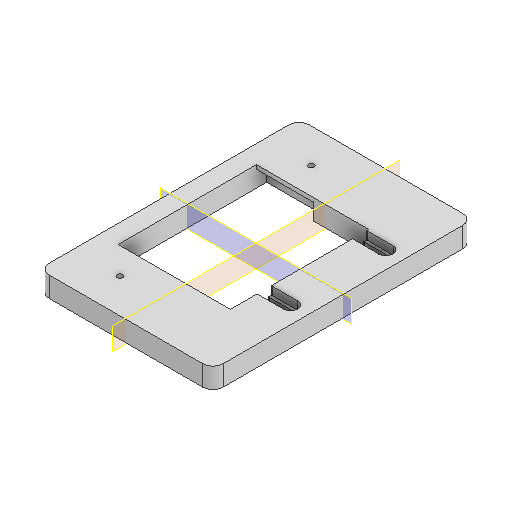
# Autodesk Inventor part: TIRFImager_base_v0
Saved by Autodesk Inventor 2022 (Build 260153000, 153)
## iProperties
Created: 2022-05-21
Part Number: TIRFImager_base_v0
Material: Generisch
Document SubType Name: Modeling
Designer: diederichbenedict
Density: 1 g/cm^3
Appearance: Vorgabe
Author: diederichbenedict
Autodesk Inventor part; units mm, degrees
ref_plane "YZ Plane" through (0, 0, 0) normal (1, 0, 0) x (0, 1, 0)
ref_plane "XZ Plane" through (0, 0, 0) normal (0, 1, 0) x (-1, 0, 0)
ref_plane "XY Plane" through (0, 0, 0) normal (0, 0, 1) x (1, 0, 0)
sketch "Skizze1" plane through (0, 0, 0) normal (0, 1, 0) x (-1, 0, 0)
  line L0 (-37.75, -63.9) -> (37.75, -63.9)
  line L1 (42.75, -58.9) -> (42.75, 58.9)
  line L2 (37.75, 63.9) -> (-37.75, 63.9)
  line L3 (-42.75, 58.9) -> (-42.75, -58.9)
  line L4 (-42.75, -63.9) -> (42.75, 63.9) construction
  line L5 (42.75, -63.9) -> (-42.75, 63.9) construction
  arc A0 (42.75, 58.9) -> (37.75, 63.9) centre (37.75, 58.9) ccw
  arc A1 (-37.75, 63.9) -> (-42.75, 58.9) centre (-37.75, 58.9) ccw
  arc A2 (-42.75, -58.9) -> (-37.75, -63.9) centre (-37.75, -58.9) ccw
  arc A3 (37.75, -63.9) -> (42.75, -58.9) centre (37.75, -58.9) ccw
  point P0 (0, 0)
  dimension "d0" = 85.5
  dimension "d1" = 127.8
  dimension "d2" = 5
  constraints: 12 end point, 8 point on circle, 8 point on line, 8 tangent, 4 centre point, 3 equal radius, 2 midpoint, 2 parallel, 1 horizontal, 1 perpendicular
  measures "d0" distance of L5.end L4.end
  measures "d1" distance of L4.end L5.start
  measures "d2" radius of A0
extrude "Extrusion1" add sketch "Skizze1" along normal blind 10
ref_plane "Arbeitsebene1" through (37.75, 0, 0) normal (0, 0, -1) x (-1, 0, 0)
ref_plane "Arbeitsebene2" through (0, 0, 58.9) normal (1, 0, 0) x (0, 0, -1)
sketch "Skizze2" plane through (0, 10, 0) normal (0, 1, 0) x (1, 0, 0)
  line L0 (-6.95, 38) -> (-32.75, 38) projected
  line L1 (-32.75, -38) -> (-6.95, -38) projected
  line L2 (-6.95, -38) -> (-6.95, -2.5) projected
  line L3 (-32.75, 38) -> (-32.75, -38) projected
  line L4 (-32.75, -38) -> (-6.95, -38)
  line L5 (-6.95, -38) -> (-6.95, 38)
  line L6 (-6.95, 38) -> (-32.75, 38)
  line L7 (-32.75, 38) -> (-32.75, -38)
  line L8 (-5.95, 39) -> (-5.95, -39)
  line L9 (-5.95, -39) -> (-33.75, -39)
  line L10 (-33.75, -39) -> (-33.75, 39)
  line L11 (-33.75, 39) -> (-5.95, 39)
  point P0 (0, 0)
  dimension "d5" = 1
  constraints: 16 end point, 4 parallel, 2 perpendicular, 1 horizontal, 3 other
  measures "d5" distance between parallel lines of L5 L8
extrude "Extrusion2" cut sketch "Skizze2" against normal through all contours L5 L2 L1 L3 L0 | L8 L9 L10 L11
ref_plane "Arbeitsebene3" through (-32.75, 5, -38) normal (0, 1, 0) x (0, 0, 1)
sketch "Skizze3" plane through (0, 10, 0) normal (0, 1, 0) x (1, 0, 0)
  line L0 (-5.95, -39) -> (-33.75, -39) projected
  line L1 (-33.75, -39) -> (-33.75, 39) projected
  line L2 (-33.75, 39) -> (-5.95, 39) projected
  line L3 (-5.95, 39) -> (-5.95, -39) projected
  arc A0 (-37.75, 63.9) -> (-42.75, 58.9) centre (-37.75, 58.9) ccw projected
  line L4 (-42.75, 58.9) -> (-42.75, -58.9) projected
  arc A1 (-42.75, -58.9) -> (-37.75, -63.9) centre (-37.75, -58.9) ccw projected
  line L5 (-37.75, -63.9) -> (37.75, -63.9) projected
  arc A2 (37.75, -63.9) -> (42.75, -58.9) centre (37.75, -58.9) ccw projected
  line L6 (42.75, -58.9) -> (42.75, 58.9) projected
  arc A3 (42.75, 58.9) -> (37.75, 63.9) centre (37.75, 58.9) ccw projected
  line L7 (37.75, 63.9) -> (-37.75, 63.9) projected
  line L8 (-33.75, -39) -> (-33.75, 39) projected
  line L9 (-5.95, 39) -> (-5.95, -39) projected
  line L10 (-33.75, -39) -> (-5.95, -39)
  line L11 (-5.95, -39) -> (-5.95, -34)
  line L12 (-5.95, -34) -> (-33.75, -34)
  line L13 (-33.75, -34) -> (-33.75, -39)
  line L14 (-33.75, 39) -> (-5.95, 39)
  line L15 (-5.95, 39) -> (-5.95, 34)
  line L16 (-5.95, 34) -> (-33.75, 34)
  line L17 (-33.75, 34) -> (-33.75, 39)
  point P0 (0, 0)
  point P1 (-5.95, 34)
  point P2 (-5.95, -34)
  dimension "d8" = 27.8
  dimension "d9" = 5
  dimension "d10" = 5
  constraints: 16 end point, 4 parallel, 2 horizontal, 2 perpendicular, 2 point on line
  measures "d8" distance of L12.end L11.end
  measures "d9" distance of L11.end L10.end
  measures "d10" distance of L14.end L15.end
extrude "Extrusion3" add sketch "Skizze3" against normal blind 1 contours L0 L1 L12 L3 | L16 L1 L2 L3
sketch "Skizze4" plane through (0, 0, 0) normal (0, -1, 0) x (1, 0, 0)
  line L0 (-33.75, 39) -> (-5.95, 39) projected
  line L1 (-5.95, 39) -> (-5.95, -39) projected
  line L2 (-5.95, -39) -> (-33.75, -39) projected
  line L3 (-33.75, -39) -> (-33.75, 39) projected
  arc A0 (-42.75, -58.9) -> (-37.75, -63.9) centre (-37.75, -58.9) ccw projected
  line L4 (37.75, -63.9) -> (-37.75, -63.9) projected
  arc A1 (37.75, -63.9) -> (42.75, -58.9) centre (37.75, -58.9) ccw projected
  line L5 (42.75, 58.9) -> (42.75, -58.9) projected
  arc A2 (42.75, 58.9) -> (37.75, 63.9) centre (37.75, 58.9) ccw projected
  line L6 (-37.75, 63.9) -> (37.75, 63.9) projected
  arc A3 (-37.75, 63.9) -> (-42.75, 58.9) centre (-37.75, 58.9) ccw projected
  line L7 (-42.75, -58.9) -> (-42.75, 58.9) projected
  line L8 (-5.95, -34) -> (-5.95, 34) projected
  line L9 (-5.95, 34) -> (21.3958, 34)
  line L10 (21.3958, 34) -> (21.3958, -34)
  line L11 (21.3958, -34) -> (-5.95, -34)
  line L12 (-5.95, -34) -> (-5.95, 34)
  line L13 (3.55, 7.5) -> (3.55, -8) projected
  point P0 (0, 0)
  point P1 (-5.95, -34)
  dimension "d14" = 5
  dimension "d15" = 5
  constraints: 8 end point, 2 parallel, 1 horizontal, 1 perpendicular, 1 point on line
  measures "d14" distance between parallel lines of L2 L11
  measures "d15" distance between parallel lines of L9 L0
extrude "Extrusion4" cut sketch "Skizze4" against normal through all contours L9 L10 L11 L1
sketch "Skizze5" plane through (0, 0, 0) normal (0, -1, 0) x (1, 0, 0)
  arc A0 (-42.75, -58.9) -> (-37.75, -63.9) centre (-37.75, -58.9) ccw projected
  line L0 (37.75, -63.9) -> (-37.75, -63.9) projected
  arc A1 (37.75, -63.9) -> (42.75, -58.9) centre (37.75, -58.9) ccw projected
  line L1 (42.75, 58.9) -> (42.75, -58.9) projected
  arc A2 (42.75, 58.9) -> (37.75, 63.9) centre (37.75, 58.9) ccw projected
  line L2 (-37.75, 63.9) -> (37.75, 63.9) projected
  arc A3 (-37.75, 63.9) -> (-42.75, 58.9) centre (-37.75, 58.9) ccw projected
  line L3 (-42.75, -58.9) -> (-42.75, 58.9) projected
  line L4 (-5.95, 34) -> (21.3958, 34) projected
  line L5 (21.3958, 34) -> (21.3958, -34) projected
  line L6 (21.3958, -34) -> (-5.95, -34) projected
  line L7 (-5.95, -34) -> (-5.95, -39) projected
  line L8 (-5.95, -39) -> (-33.75, -39) projected
  line L9 (-33.75, -39) -> (-33.75, 39) projected
  line L10 (-33.75, 39) -> (-5.95, 39) projected
  line L11 (-5.95, 39) -> (-5.95, 34) projected
  circle A4 centre (-19.85, -47) radius 1.4
  circle A5 centre (-19.85, 47) radius 1.4
  point P0 (0, 0)
  dimension "d18" = 2.8
  dimension "d19" = 2.8
  dimension "d20" = 8
  dimension "d21" = 8
  constraints: 2 centre point
  measures "d18" diameter of A4
  measures "d19" diameter of A5
  measures "d20" distance from line of L8 A4.centre
  measures "d21" distance from line of A5.centre L10
extrude "Extrusion5" cut sketch "Skizze5" against normal through all contours A4 | A5
sketch "Skizze6" plane through (0, 10, 0) normal (0, 1, 0) x (1, 0, 0)
  circle A0 centre (25.45, -17.36) radius 1.57 projected
  circle A1 centre (32.55, -17.36) radius 1.57 projected
  circle A2 centre (32.55, 29.54) radius 1.57 projected
  circle A3 centre (25.45, 29.54) radius 1.57 projected
  line L0 (21.45, 51.1) -> (36.55, 51.1) projected
  line L1 (36.55, 42.04) -> (36.55, 51.1) projected
  line L2 (34.55, 42.04) -> (36.55, 42.04) projected
  line L3 (34.55, 34.04) -> (34.55, 42.04) projected
  line L4 (36.55, 34.04) -> (34.55, 34.04) projected
  line L5 (36.55, -21.86) -> (36.55, 34.04) projected
  line L6 (36.55, -21.86) -> (34.55, -21.86) projected
  line L7 (34.55, -21.86) -> (34.55, -29.86) projected
  line L8 (34.55, -29.86) -> (36.55, -29.86) projected
  line L9 (36.55, -29.86) -> (36.55, -38.92) projected
  line L10 (36.55, -38.92) -> (21.45, -38.92) projected
  line L11 (21.45, -38.92) -> (21.45, -29.86) projected
  line L12 (21.45, -29.86) -> (23.45, -29.86) projected
  line L13 (23.45, -29.86) -> (23.45, -21.86) projected
  line L14 (23.45, -21.86) -> (21.45, -21.86) projected
  line L15 (21.45, -21.86) -> (21.45, 34.04) projected
  line L16 (23.45, 34.04) -> (21.45, 34.04) projected
  line L17 (23.45, 42.04) -> (23.45, 34.04) projected
  line L18 (21.45, 42.04) -> (23.45, 42.04) projected
  line L19 (21.45, 51.1) -> (21.45, 42.04) projected
  circle A4 centre (25.45, 29.54) radius 1.57
  circle A5 centre (32.55, 29.54) radius 1.57
  circle A6 centre (25.45, -17.36) radius 1.57
  circle A7 centre (32.55, -17.36) radius 1.57
  circle A8 centre (21.9, 29.54) radius 1.57
  circle A9 centre (29, 29.54) radius 1.57
  circle A10 centre (21.9, -17.36) radius 1.57
  circle A11 centre (29, -17.36) radius 1.57
  point P0 (0, 0)
  constraints: 8 centre point, 4 coincident, 4 concentric
hole "Bohrung1" at (29, 10, 17.36) at (29, 10, -29.54) at (21.9, 10, -29.54) at (21.9, 10, 17.36) direction (0, -1, 0) diameter 4 end through all counterbore diameter 7 counterbore depth 4
sketch "Skizze7" plane through (21.9, 6, -29.54) normal (0, 1, 0) x (1, 0, 0)
  circle A0 centre (7.1, 0) radius 2 projected
  arc A1 (-0.5042, -1.9354) -> (-0.5042, 1.9354) centre (0, 0) ccw projected
  line L0 (9.2, -49.54) -> (5, -49.54) projected
  circle A2 centre (7.1, -46.9) radius 2 projected
  arc A3 (-0.5042, -48.8354) -> (-0.5042, -44.9646) centre (0, -46.9) ccw projected
  arc A4 (-0.5042, -50.3635) -> (-0.5042, -43.4365) centre (0, -46.9) ccw projected
  line L1 (0, -46.9) -> (10.0593, -46.9) construction
  line L2 (0, -44.9) -> (10.0593, -44.9)
  line L3 (10.0593, -48.9) -> (0, -48.9)
  arc A5 (0, -44.9) -> (0, -48.9) centre (0, -46.9) ccw
  arc A6 (10.0593, -48.9) -> (10.0593, -44.9) centre (10.0593, -46.9) ccw
  arc A7 (-0.5042, -1.9354) -> (-0.5042, 1.9354) centre (0, 0) ccw projected
  line L4 (0, 0) -> (10.0593, 0) construction
  line L5 (0, 2) -> (10.0593, 2)
  line L6 (10.0593, -2) -> (0, -2)
  arc A8 (0, 2) -> (0, -2) centre (0, 0) ccw
  arc A9 (10.0593, -2) -> (10.0593, 2) centre (10.0593, 0) ccw
  point P0 (-21.9, -29.54)
  point P1 (5.0296, -46.9)
  point P2 (5.0296, 0)
  point P3 (0, -48.9)
  point P4 (0, -2)
  point P5 (0, 2)
  constraints: 16 end point, 8 point on circle, 8 tangent, 4 centre point, 3 parallel, 2 midpoint, 1 horizontal
extrude "Extrusion6" cut sketch "Skizze7" against normal through all
sketch "Skizze8" plane through (0, 10, 0) normal (0, 1, 0) x (1, 0, 0)
  arc A0 (21.3958, 26.0765) -> (21.3958, 33.0035) centre (21.9, 29.54) ccw projected
  line L0 (21.3958, 26.0765) -> (21.3958, -13.8965) projected
  arc A1 (21.3958, -20.8235) -> (21.3958, -13.8965) centre (21.9, -17.36) ccw projected
  line L1 (21.3958, -20.8235) -> (21.3958, -34) projected
  line L2 (21.3958, -34) -> (-33.75, -34) projected
  line L3 (-33.75, -34) -> (-33.75, 34) projected
  line L4 (-33.75, 34) -> (21.3958, 34) projected
  line L5 (21.3958, 34) -> (21.3958, 33.0035) projected
  circle A2 centre (29, -17.36) radius 3.5 projected
  circle A3 centre (29, 29.54) radius 3.5 projected
  circle A4 centre (-19.85, -47) radius 1.4 projected
  circle A5 centre (-19.85, 47) radius 1.4 projected
  arc A6 (-37.75, 63.9) -> (-42.75, 58.9) centre (-37.75, 58.9) ccw projected
  line L6 (-42.75, 58.9) -> (-42.75, -58.9) projected
  arc A7 (-42.75, -58.9) -> (-37.75, -63.9) centre (-37.75, -58.9) ccw projected
  line L7 (-37.75, -63.9) -> (37.75, -63.9) projected
  arc A8 (37.75, -63.9) -> (42.75, -58.9) centre (37.75, -58.9) ccw projected
  line L8 (42.75, -58.9) -> (42.75, 58.9) projected
  arc A9 (42.75, 58.9) -> (37.75, 63.9) centre (37.75, 58.9) ccw projected
  line L9 (37.75, 63.9) -> (-37.75, 63.9) projected
  arc A10 (21.3958, 26.0765) -> (21.3958, 33.0035) centre (21.9, 29.54) ccw projected
  line L10 (21.9, 29.54) -> (34.3149, 29.54) construction
  line L11 (21.9, 26.04) -> (34.3149, 26.04)
  line L12 (34.3149, 33.04) -> (21.9, 33.04)
  arc A11 (21.9, 33.04) -> (21.9, 26.04) centre (21.9, 29.54) ccw
  arc A12 (34.3149, 26.04) -> (34.3149, 33.04) centre (34.3149, 29.54) ccw
  line L13 (21.9, -17.36) -> (34.3149, -17.36) construction
  line L14 (21.9, -20.86) -> (34.3149, -20.86)
  line L15 (34.3149, -13.86) -> (21.9, -13.86)
  arc A13 (21.9, -13.86) -> (21.9, -20.86) centre (21.9, -17.36) ccw
  arc A14 (34.3149, -20.86) -> (34.3149, -13.86) centre (34.3149, -17.36) ccw
  point P0 (0, 0)
  point P1 (28.1075, 29.54)
  point P2 (28.1075, -17.36)
  point P3 (21.3958, -13.8965)
  point P4 (21.3958, 33.0035)
  constraints: 16 end point, 8 point on circle, 8 tangent, 4 centre point, 3 parallel, 2 midpoint, 1 horizontal
extrude "Extrusion7" cut sketch "Skizze8" against normal up to surface (4 mm away) contours A11 A0 | A0 L12 A3 L11 | A1 A13 | A3 | A3 L12 A12 L11 | L15 A2 L14 A1 | L15 A14 L14 A2 | A2
sketch "Skizze9" plane through (0, 9, 0) normal (0, -1, 0) x (1, 0, 0)
  circle A0 centre (-19.85, 47) radius 1.4 projected
  circle A1 centre (-19.85, -47) radius 1.4 projected
  arc A2 (-42.75, -58.9) -> (-37.75, -63.9) centre (-37.75, -58.9) ccw projected
  line L0 (37.75, -63.9) -> (-37.75, -63.9) projected
  arc A3 (37.75, -63.9) -> (42.75, -58.9) centre (37.75, -58.9) ccw projected
  line L1 (42.75, 58.9) -> (42.75, -58.9) projected
  arc A4 (42.75, 58.9) -> (37.75, 63.9) centre (37.75, 58.9) ccw projected
  line L2 (-37.75, 63.9) -> (37.75, 63.9) projected
  arc A5 (-37.75, 63.9) -> (-42.75, 58.9) centre (-37.75, 58.9) ccw projected
  line L3 (-42.75, -58.9) -> (-42.75, 58.9) projected
  line L4 (21.9, 19.36) -> (31.9593, 19.36) projected
  arc A6 (31.9593, 15.36) -> (31.9593, 19.36) centre (31.9593, 17.36) ccw projected
  line L5 (31.9593, 15.36) -> (21.9, 15.36) projected
  arc A7 (21.3958, 15.4246) -> (21.9, 15.36) centre (21.9, 17.36) ccw projected
  line L6 (21.3958, 15.4246) -> (21.3958, -27.6046) projected
  arc A8 (21.9, -27.54) -> (21.3958, -27.6046) centre (21.9, -29.54) ccw projected
  line L7 (21.9, -27.54) -> (31.9593, -27.54) projected
  arc A9 (31.9593, -31.54) -> (31.9593, -27.54) centre (31.9593, -29.54) ccw projected
  line L8 (31.9593, -31.54) -> (21.9, -31.54) projected
  arc A10 (21.3958, -31.4754) -> (21.9, -31.54) centre (21.9, -29.54) ccw projected
  line L9 (21.3958, -31.4754) -> (21.3958, -34) projected
  line L10 (21.3958, -34) -> (-5.95, -34) projected
  line L11 (-5.95, -34) -> (-5.95, -39) projected
  line L12 (-5.95, -39) -> (-33.75, -39) projected
  line L13 (-33.75, -39) -> (-33.75, 39) projected
  line L14 (-33.75, 39) -> (-5.95, 39) projected
  line L15 (-5.95, 39) -> (-5.95, 34) projected
  line L16 (-5.95, 34) -> (21.3958, 34) projected
  line L17 (21.3958, 34) -> (21.3958, 19.2954) projected
  arc A11 (21.9, 19.36) -> (21.3958, 19.2954) centre (21.9, 17.36) ccw projected
  line L18 (-33.75, 39) -> (-5.95, 39) projected
  line L19 (-33.75, 39) -> (-5.95, 39)
  line L20 (-5.95, 39) -> (-5.95, 34)
  line L21 (-5.95, 34) -> (-33.75, 34)
  line L22 (-33.75, 34) -> (-33.75, 39)
  line L23 (-5.95, -39) -> (-33.75, -39) projected
  line L24 (-33.75, -39) -> (-33.75, -34) projected
  line L25 (-5.95, -39) -> (-33.75, -39)
  line L26 (-33.75, -39) -> (-33.75, -34)
  line L27 (-33.75, -34) -> (-5.95, -34)
  line L28 (-5.95, -34) -> (-5.95, -39)
  point P0 (0, 0)
  constraints: 16 end point, 4 parallel, 2 horizontal, 2 perpendicular
extrude "Extrusion8" add sketch "Skizze9" along normal blind 1 contours L21 L13 L14 L15 | L27 L11 L12 L13
